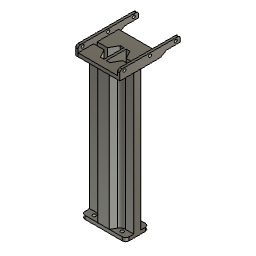
arm_long_v1 (Autodesk Fusion 360 design; units mm, degrees)
Autodesk Fusion 360 part; units mm, degrees
note: some values were not read from the file. Set by a fixed rule: which face or edge a step refers to.
sketch "스케치1" plane through (0, 0, 0) normal (0, 0, 1) x (1, 0, 0)
  line L0 (0, 0) -> (38, 0)
  line L1 (38, 0) -> (38, 20)
  line L2 (38, 20) -> (0, 20)
  line L3 (0, 20) -> (0, 0)
  line L4 (0, 0) -> (0, 10)
  circle A0 centre (7, 16) radius 1.5
  circle A1 centre (31, 16) radius 1.5
  circle A2 centre (7, 4) radius 1.5
  circle A3 centre (31, 4) radius 1.5
  circle A4 centre (19, 10) radius 4
  line L5 (0, 10) -> (0, 13)
  line L6 (0, 13) -> (10, 13)
  line L7 (10, 13) -> (14.041452, 20)
  line L8 (10, 13) -> (18.082904, 13) construction
  line L9 (0, 10) -> (0, 7)
  line L10 (0, 10) -> (0, 7)
  line L11 (0, 7) -> (10, 7)
  line L12 (10, 7) -> (14.031129, 0.01788)
  line L13 (38, 10) -> (38, 13)
  line L14 (38, 13) -> (28, 13)
  line L15 (28, 13) -> (23.958548, 20)
  line L16 (28, 13) -> (36.082904, 13) construction
  line L17 (23.958548, 20) -> (14.041452, 20)
  line L18 (38, 10) -> (38, 7)
  line L19 (38, 7) -> (28, 7)
  line L20 (28, 7) -> (23.958549, 0)
  line L21 (28, 7) -> (36.082904, 7) construction
  line L22 (14.041452, 20) -> (23.958548, 20)
  line L23 (14.031129, 0.01788) -> (23.958549, 0)
  line L24 (27.133975, 11.5) -> (23.092523, 18.5)
  line L25 (14.907477, 18.5) -> (23.092523, 18.5)
  line L26 (10.866026, 11.5) -> (14.907477, 18.5)
  line L27 (1.5, 11.5) -> (10.866026, 11.5)
  line L28 (1.5, 10) -> (1.5, 11.5)
  line L29 (1.5, 10) -> (1.5, 8.5)
  line L30 (1.5, 8.5) -> (10.866026, 8.5)
  line L31 (10.866026, 8.5) -> (14.898055, 1.516321)
  line L32 (14.898055, 1.516321) -> (23.093424, 1.501561)
  line L33 (27.133975, 8.5) -> (23.093424, 1.501561)
  line L34 (36.5, 8.5) -> (27.133975, 8.5)
  line L35 (36.5, 10) -> (36.5, 8.5)
  line L36 (36.5, 10) -> (36.5, 11.5)
  line L37 (36.5, 11.5) -> (27.133975, 11.5)
  line L38 (19, 18.5) -> (20, 18.5)
  line L39 (19, 18.5) -> (18, 18.5)
  line L40 (18, 18.5) -> (17.969402, 1.510789)
  line L41 (20, 18.5) -> (19.969395, 1.507187)
  dimension "d1" = 38
  dimension "d2" = 20
  dimension "d7" = 3
  dimension "d8" = 3
  dimension "d9" = 3
  dimension "d10" = 3
  dimension "d11" = 8
  dimension "d12" = 3
  dimension "d13" = 10
  dimension "d14" = 60
  dimension "d15" = 120
  dimension "d16" = 10
  dimension "d17" = 120
  dimension "d19" = 10
  dimension "d20" = 120
  dimension "d21" = 1.5
  dimension "d22" = 1
  dimension "d23" = 1
  constraint horizontal L0
  constraint vertical L1
  constraint horizontal L2
  constraint vertical L3
  constraint coincident L0.start L3.end
  constraint midpoint L3 L4.end
  constraint midpoint L1 L13.start
  constraint horizontal L6
  constraint horizontal L8
  constraint coincident L4 L9.end
  constraint coincident L1 L13.end
  constraint perpendicular L1 L14
  constraint horizontal L16
  constraint horizontal L19
  constraint horizontal L21
  constraint midpoint L25 L38.start
  constraint horizontal L39
  constraint perpendicular L32 L40
  constraint perpendicular L32 L41
  measures "d1" distance of L0.start L0.end
  measures "d2" distance of L0.start L2.end
  measures "d7" diameter of A0
  measures "d8" diameter of A1
  measures "d9" diameter of A2
  measures "d10" diameter of A3
  measures "d11" diameter of A4
  measures "d12" distance of L4.end L5.end
  measures "d13" distance of L5.end L6.end
  measures "d14" angle of L7 L8
  measures "d15" angle of L11 L12
  measures "d16" distance of L13.end L14.end
  measures "d17" angle of L15 L16
  measures "d19" distance of L18.end L19.end
  measures "d20" angle of L20 L21
  measures "d22" distance of L38.start L38.end
  measures "d23" distance of L38.start L39.end
extrude "돌출1" add sketch "스케치1" along normal blind 3 contours L0 L3 L4 L11 L12 L23 | L0 L1 L19 L20 | L1 L2 L3 L4 L5 L6 L7 L9 L10 L11 L12 L13 L14 L15 L17 L18 L19 L20 L22 L23 | L2 L3 L6 L7 | L1 L2 L14 L15 | A0 | A1 | A2 | A3 | A4 L41 | A4 L24 L25 L32 L33 L34 L35 L36 L37 L41 | A4 L40 L41 | A4 L25 L38 L39 L40 L41 | A4 L32 L40 L41 | A4 L40 | A4 L25 L26 L27 L28 L29 L30 L31 L32 L40 picked at (1.838918, 3.592146) picked at (36.161082, 3.592146) picked at (19, 19.5) picked at (1.838918, 16.407854) picked at (36.161082, 16.407855) picked at (6.622111, 16.698578) picked at (31.416042, 16.557028) picked at (6.515471, 3.740367) picked at (31.383155, 4.412943) picked at (21.367256, 10.890684) picked at (24.064476, 5.772594) picked at (19.320346, 11.289091) picked at (18.495814, 16.989008) picked at (18.971927, 3.006014) picked at (17.212157, 10.738455) picked at (13.932618, 14.22437) makes body 1
extrude "돌출2" add sketch "스케치1" against normal blind 2.5 contours A4 L41 | A4 L40 L41 | A4 L40 picked at (21.367256, 10.890684) picked at (19.320346, 11.289091) picked at (17.212157, 10.738455) bodies 1
extrude "돌출3" cut sketch "스케치1" along normal blind 3 contours A0 | A1 | A2 | A3 picked at (6.622111, 16.698578) picked at (31.416042, 16.557028) picked at (6.515471, 3.740367) picked at (31.383155, 4.412943) bodies 1
extrude "돌출4" add sketch "스케치1" along normal blind 123 contours L1 L2 L3 L4 L5 L6 L7 L9 L10 L11 L12 L13 L14 L15 L17 L18 L19 L20 L22 L23 | A4 L40 L41 | A4 L25 L38 L39 L40 L41 | A4 L32 L40 L41 picked at (19, 19.5) picked at (19.320346, 11.289091) picked at (18.495814, 16.989008) picked at (18.971927, 3.006014) bodies 1
sketch "스케치2" plane through (0, 0, 123) normal (0, 0, 1) x (-1, 0, 0)
  line L0 (-36.5, -11.5) -> (-36.5, -8.5)
  line L1 (-36.5, -8.5) -> (-27.133975, -8.5)
  line L2 (-27.133975, -8.5) -> (-23.093424, -1.501561)
  line L3 (-23.093424, -1.501561) -> (-19.969395, -1.507187)
  line L4 (-19.969395, -1.507187) -> (-20, -18.5)
  line L5 (-20, -18.5) -> (-23.092523, -18.5)
  line L6 (-23.092523, -18.5) -> (-27.133975, -11.5)
  line L7 (-27.133975, -11.5) -> (-36.5, -11.5)
  line L8 (-1.5, -8.5) -> (-1.5, -11.5)
  line L9 (-1.5, -11.5) -> (-10.866026, -11.5)
  line L10 (-10.866026, -11.5) -> (-14.907477, -18.5)
  line L11 (-14.907477, -18.5) -> (-18, -18.5)
  line L12 (-18, -18.5) -> (-17.969402, -1.510789)
  line L13 (-17.969402, -1.510789) -> (-14.898055, -1.516321)
  line L14 (-14.898055, -1.516321) -> (-10.866026, -8.5)
  line L15 (-10.866026, -8.5) -> (-1.5, -8.5)
  line L16 (0, -13) -> (0, -7)
  line L17 (0, -7) -> (-10, -7)
  line L18 (-10, -7) -> (-14.031129, -0.01788)
  line L19 (-14.031129, -0.01788) -> (-23.958549, 0)
  line L20 (-23.958549, 0) -> (-28, -7)
  line L21 (-28, -7) -> (-38, -7)
  line L22 (-38, -7) -> (-38, -13)
  line L23 (-38, -13) -> (-28, -13)
  line L24 (-28, -13) -> (-23.958548, -20)
  line L25 (-23.958548, -20) -> (-14.041452, -20)
  line L26 (-14.041452, -20) -> (-10, -13)
  line L27 (-10, -13) -> (0, -13)
  line L28 (-18.994839, -0.00894) -> (-1.994866, -0.039558)
  line L29 (-1.994866, -0.039558) -> (-1.985861, 4.960426)
  line L30 (-1.985861, 4.960426) -> (-35.985861, 4.960426)
  line L31 (-35.985861, 4.960426) -> (-35.985861, -56.039574)
  line L32 (-35.985861, -56.039574) -> (-1.985861, -56.039574)
  line L33 (-1.985861, -56.039574) -> (-1.985861, 4.960426)
  line L34 (-35.985861, 4.960426) -> (-37.985861, 4.960426)
  line L35 (-1.985861, 4.960426) -> (0.014139, 4.960426)
  line L36 (0.014139, 4.960426) -> (0.014139, -56.039574)
  line L37 (0.014139, -56.039574) -> (-1.985861, -56.039574)
  line L38 (-1.985861, -56.039574) -> (-1.985861, 4.960426)
  line L39 (-37.985861, 4.960426) -> (-35.985861, 4.960426)
  line L40 (-35.985861, 4.960426) -> (-35.985861, -56.039574)
  line L41 (-35.985861, -56.039574) -> (-37.985861, -56.039574)
  line L42 (-37.985861, -56.039574) -> (-37.985861, 4.960426)
  line L43 (-1.994866, -0.039558) -> (-2.030888, -20.039526)
  line L44 (-2.030888, -20.039526) -> (-2.030888, -30.039526)
  line L45 (-2.030888, -30.039526) -> (-36.030888, -30.039526)
  line L46 (-35.985861, -56.039574) -> (-35.985861, -47.039574)
  line L47 (-35.985861, -47.039574) -> (-37.985861, -47.039574)
  line L48 (-35.985861, -47.039574) -> (0.014139, -47.039574)
  line L49 (-36.030888, -30.039526) -> (-38.030888, -30.039526)
  line L50 (-2.030888, -30.039526) -> (-0.030888, -30.039526)
  dimension "d32" = 17
  dimension "d33" = 5
  dimension "d34" = 34
  dimension "d35" = 61
  dimension "d36" = 2
  dimension "d37" = 2
  dimension "d38" = 61
  dimension "d39" = 20
  dimension "d40" = 10
  dimension "d41" = 34
  dimension "d56" = 9
  dimension "d57" = 36
  dimension "d60" = 2
  dimension "d61" = 2
  constraint parallel L19 L28
  constraint perpendicular L28 L29
  constraint horizontal L30
  constraint vertical L31
  constraint horizontal L32
  constraint vertical L33
  constraint perpendicular L31 L34
  constraint horizontal L35
  constraint vertical L36
  constraint horizontal L37
  constraint vertical L38
  constraint horizontal L39
  constraint vertical L40
  constraint horizontal L41
  constraint vertical L42
  constraint perpendicular L28 L43
  constraint perpendicular L37 L44
  constraint perpendicular L40 L45
  constraint perpendicular L41 L46
  constraint perpendicular L42 L47
  constraint perpendicular L36 L48
  constraint perpendicular L42 L49
  constraint perpendicular L36 L50
extrude "돌출5" add sketch "스케치2" along normal blind 3 separate body contours L0 L1 L7 L21 L23 L31 L40 L42 | L0 L1 L7 L31 L40 | L1 L2 L3 L4 L5 L6 L7 L31 L40 | L1 L2 L3 L4 L5 L6 L7 L9 L10 L11 L12 L13 L14 L15 L17 L18 L19 L20 L21 L23 L24 L25 L26 L27 L28 L31 L40 L43 | L23 L31 L40 L42 L45 L49 | L23 L24 L25 L26 L27 L31 L40 L43 L44 L45 | L19 L20 L21 L28 L29 L30 L31 L40 | L21 L31 L34 L39 L40 L42 | L31 L33 L38 L40 L45 L48 L50 | L31 L40 L42 L45 L47 L49 | L31 L32 L33 L38 L40 L46 L48 | L31 L40 L41 L42 L46 L47 | L27 L33 L38 L43 L44 L50 | L16 L17 L27 L33 L35 L36 L38 L48 | L33 L36 L37 L38 L48 | L17 L18 L28 L43 | L8 L9 L15 L16 L17 L27 L33 L38 | L8 L9 L15 L33 L38 | L9 L10 L11 L12 L13 L14 L15 L43 picked at (-37.490574, -10.5) picked at (-36.32862, -9.5) picked at (-22.36779, -10.502396) picked at (-19.323132, -12.835729) picked at (-36.667537, -18.679842) picked at (-20.658432, -26.693017) picked at (-29.314803, -0.679858) picked at (-36.652528, -3.013191) picked at (-13.334203, -41.372891) picked at (-36.667537, -41.372891) picked at (-13.319194, -53.039574) picked at (-37.319194, -50.039574) picked at (-2.00087, -21.02635) picked at (-0.657241, -30.026367) picked at (-1.319194, -50.039574) picked at (-8.675332, -2.352479) picked at (-0.5, -10.5) picked at (-1.823907, -9.5) picked at (-15.611809, -10.503596) makes body 2
extrude "돌출6" cut sketch "스케치2" along normal blind 3 contours L31 L33 L38 L40 L45 L48 L50 | L31 L32 L33 L38 L40 L46 L48 | L27 L33 L38 L43 L44 L50 picked at (-13.334203, -41.372891) picked at (-13.319194, -53.039574) picked at (-2.00087, -21.02635) bodies 2
sketch "스케치3" plane through (37.985861, 0, 0) normal (1, 0, 0) x (0, 1, 0)
  line L0 (-4.960426, 123) -> (56.039574, 123)
  line L1 (56.039574, 123) -> (56.039574, 126)
  line L2 (56.039574, 126) -> (-4.960426, 126)
  line L3 (-4.960426, 126) -> (-4.960426, 123)
  line L4 (-4.960426, 126) -> (-4.960426, 131)
  line L5 (-4.960426, 126) -> (-4.960426, 128.8)
  line L6 (-4.960426, 131) -> (56.039574, 131)
  line L7 (56.039574, 131) -> (56.039574, 126)
  line L8 (56.039574, 126) -> (-4.960426, 126)
  line L9 (-4.960426, 126) -> (-4.960426, 131)
  line L10 (-4.960426, 128.8) -> (56.039574, 128.8)
  line L11 (-4.960426, 128.8) -> (-0.960426, 128.8)
  line L12 (-0.960426, 128.8) -> (21.039574, 128.8)
  line L13 (21.039574, 128.8) -> (43.039574, 128.8)
  circle A0 centre (-0.960426, 128.8) radius 1.3
  circle A1 centre (21.039574, 128.8) radius 1.3
  circle A2 centre (43.039574, 128.8) radius 1.3
  line L14 (43.039574, 128.8) -> (47.039574, 128.8)
  line L15 (47.039574, 128.8) -> (47.039574, 131)
  line L16 (47.039574, 128.8) -> (47.039574, 126.000002)
  line L17 (-4.960426, 123) -> (30.039574, 123)
  line L18 (30.039574, 123) -> (35.235727, 126)
  line L19 (30.039574, 123) -> (36.039574, 123) construction
  dimension "d46" = 5
  dimension "d47" = 2.8
  dimension "d48" = 61
  dimension "d49" = 4
  dimension "d50" = 22
  dimension "d51" = 22
  dimension "d52" = 2.6
  dimension "d53" = 2.6
  dimension "d54" = 2.6
  dimension "d55" = 4
  dimension "d62" = 35
  dimension "d63" = 30
  constraint perpendicular L2 L4
  constraint perpendicular L2 L5
  constraint horizontal L6
  constraint vertical L7
  constraint horizontal L8
  constraint vertical L9
  constraint horizontal L10
  constraint perpendicular L5 L11
  constraint horizontal L12
  constraint horizontal L13
  constraint parallel L10 L14
  constraint perpendicular L6 L15
  constraint perpendicular L8 L16
  constraint horizontal L17
  constraint horizontal L19
  measures "d52" diameter of A0
  measures "d53" diameter of A1
  measures "d54" diameter of A2
  measures "d63" angle of L18 L19
extrude "돌출7" cut sketch "스케치2" along normal blind 3 contours L31 L32 L33 L38 L40 L46 L48 | L31 L40 L41 L42 L46 L47 | L33 L36 L37 L38 L48 picked at (-13.319194, -53.039574) picked at (-37.319194, -50.039574) picked at (-1.319194, -50.039574) bodies 2
extrude "돌출8" add sketch "스케치3" against normal blind 2 separate body contours L2 L4 L5 L8 L9 L10 L11 L12 L13 A0 A1 A2 L14 L16 | L4 L6 L9 L10 L11 L12 L13 A0 A1 A2 L14 L15 picked at (33.104958, 127.866667) picked at (46.096661, 129.72135) makes body 3
copy_body "CopyPasteBodies1" bodies 3 makes body 4
move_body "이동1" bodies 4 to x (1, 0, 0) y (0, 1, 0) z (0, 0, 1) at (-36, 0, 0)
extrude "돌출9" cut sketch "스케치3" against normal blind 38 contours L0 L1 L2 L8 L18 picked at (44.372908, 124) bodies 2
extrude "돌출10" cut sketch "스케치2" along normal blind 3 contours L1 L2 L3 L4 L5 L6 L7 L31 L40 | L9 L10 L11 L12 L13 L14 L15 L43 picked at (-22.36779, -10.502396) picked at (-15.611809, -10.503596) bodies 2
thread "스레드1" "ISO Metric profile 3.5 M3.5x0.6 6H" major diameter 3.5995 minor diameter 2.93 pitch 0.6 angle 60 resizes the face on face at (32.498136, 3.925231, 2) on bodies 1
thread "스레드2" "ISO Metric profile 3.5 M3.5x0.6 6H" major diameter 3.5995 minor diameter 2.93 pitch 0.6 angle 60 resizes the face on face at (32.195699, 16.905707, 2) on bodies 1
thread "스레드3" "ISO Metric profile 3.5 M3.5x0.6 6H" major diameter 3.5995 minor diameter 2.93 pitch 0.6 angle 60 resizes the face on face at (8.498135, 3.925231, 2) on bodies 1
thread "스레드4" "ISO Metric profile 3.5 M3.5x0.6 6H" major diameter 3.5995 minor diameter 2.93 pitch 0.6 angle 60 resizes the face on face at (8.498135, 15.925231, 2) on bodies 1
extrude "돌출11" cut 1 faces at (20.218801, 8.869118, -2.5) along direction (0, 0, 1) blind 2.5 on bodies 1 bodies 1
thread "스레드5" "ISO Metric profile 3.0 M3x0.5 6H" major diameter 3.086 minor diameter 2.529 pitch 0.5 angle 60 resizes the face on face at (37.319194, -2.25881, 128.7352) on face at (36.652528, 0.237493, 129.304965) on bodies 3
thread "스레드6" "ISO Metric profile 3.0 M3x0.5 6H" major diameter 3.086 minor diameter 2.529 pitch 0.5 angle 60 resizes the face on face at (37.319194, 22.237493, 129.304965) on bodies 3
thread "스레드7" "ISO Metric profile 3.0 M3x0.5 6H" major diameter 3.086 minor diameter 2.529 pitch 0.5 angle 60 resizes the face on face at (36.652528, 44.261175, 129.244626) on bodies 3
thread "스레드8" "ISO Metric profile 3.0 M3x0.5 6H" major diameter 3.086 minor diameter 2.529 pitch 0.5 angle 60 resizes the face on face at (1.319194, 41.74119, 128.7352) on face at (0.652528, 44.237493, 129.304965) on bodies 4
thread "스레드9" "ISO Metric profile 3.0 M3x0.5 6H" major diameter 3.086 minor diameter 2.529 pitch 0.5 angle 60 resizes the face on face at (1.319194, 22.237493, 129.304965) on bodies 4
thread "스레드10" "ISO Metric profile 3.0 M3x0.5 6H" major diameter 3.086 minor diameter 2.529 pitch 0.5 angle 60 resizes the face on face at (1.319194, -2.158345, 129.304965) on bodies 4
fillet "모깎기1" radius 3 4 edges at (38, 0, 1.5) (38, 20, 1.5) (0, 0, 1.5) (0, 20, 1.5) on bodies 1
fillet "모깎기2" radius 5 4 edges at (28, 13, 63) (10, 13, 63) (10, 7, 63) (28, 7, 63) on bodies 1
combine "결합1" operation add target body 1 tool bodies 3 2 4
fillet "모깎기3" radius 2 4 edges at (0.985861, -4.960426, 131) (36.985861, -4.960426, 131) (0.985861, 47.039574, 131) (36.985861, 47.039574, 131) on bodies 1
